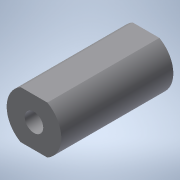
# Autodesk Inventor part: SP35V1 Vastago Cierre
Saved by Autodesk Inventor 2021.2 (Build 252289000, 289)
## iProperties
Created: 2026-08-18
Part Number: SP35V1 Vastago Cierre
Material: Generic
Document SubType Name: Modeling
Designer: nelso
Density: 1 g/cm^3
Appearance: Default
Author: nelso
Autodesk Inventor part; units mm, degrees
ref_plane "YZ Plane" through (0, 0, 0) normal (1, 0, 0) x (0, 1, 0)
ref_plane "XZ Plane" through (0, 0, 0) normal (0, 1, 0) x (-1, 0, 0)
ref_plane "XY Plane" through (0, 0, 0) normal (0, 0, 1) x (1, 0, 0)
sketch "Sketch1" plane through (0, 0, 0) normal (0, 1, 0) x (-1, 0, 0)
  circle A0 centre (0, 0) radius 9.75
  line L0 (-9.75, -8.5) -> (9.75, -8.5)
  line L1 (9.75, -8.5) -> (9.75, 8.5)
  line L2 (9.75, 8.5) -> (-9.75, 8.5)
  line L3 (-9.75, 8.5) -> (-9.75, -8.5)
  line L4 (-9.75, -8.5) -> (9.75, 8.5) construction
  line L5 (9.75, -8.5) -> (-9.75, 8.5) construction
  point P0 (4.7762, 8.5)
  point P1 (-4.7762, 8.5)
  point P2 (-4.7762, -8.5)
  point P3 (4.7762, -8.5)
  dimension "d18" = 19.5
  dimension "d19" = 17
  constraints: 12 end point, 2 midpoint, 2 parallel, 1 centre point, 1 horizontal, 1 perpendicular
  measures "d18" diameter of A0
  measures "d19" distance of L1.end L0.end
extrude "Extrusion1" add sketch "Sketch1" along normal mid plane 40 contours A0 L0 L2
sketch "Sketch2" plane through (0, 20, 0) normal (0, 1, 0) x (1, 0, 0)
  point P0 (0, 0)
hole "Hole1" at (0, 20, 0) direction (0, -1, 0) diameter 6.6 depth 10 tip angle 118 clearance for "Countersunk Flat Head Screw ISO 2009/7046" size "M6" standard "ISO"
sketch "Sketch3" plane through (0, -20, 0) normal (0, -1, 0) x (1, 0, 0)
  point P0 (0, 0)
hole "Hole2" at (0, -20, 0) direction (0, 1, 0) diameter 6.6 depth 10 tip angle 118 clearance for "Countersunk Flat Head Screw ISO 2009/7046" size "M6" standard "ISO"
body "Solid1"
